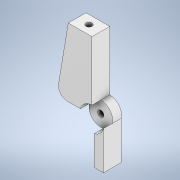
# Autodesk Inventor part: pliers
Saved by Autodesk Inventor 2020 (Build 240168000, 168)
## iProperties
Created: 2019-12-24
Part Number: pliers
Material: ABS Plastic
Document SubType Name: Modeling
Designer: metal
Density: 1.06 g/cm^3
Appearance: Smooth - White
Author: metal
Autodesk Inventor part; units mm, degrees
ref_plane "YZ Plane" through (0, 0, 0) normal (1, 0, 0) x (0, 1, 0)
ref_plane "XZ Plane" through (0, 0, 0) normal (0, 1, 0) x (-1, 0, 0)
ref_plane "XY Plane" through (0, 0, 0) normal (0, 0, 1) x (1, 0, 0)
sketch "Sketch1" plane through (0, 0, 0) normal (0, 0, 1) x (1, 0, 0)
  circle A0 centre (0, 0) radius 4
  line L0 (0, 24) -> (-8, 24)
  line L1 (0, 24) -> (0, 4)
  line L2 (-11.873, 1) -> (-3.873, 1)
  line L3 (-11.873, 1) -> (-8, 24)
  dimension "d0" = 8
  dimension "d6" = 8
  dimension "d60" = 20
  dimension "d61" = 8
  constraints: 8 end point, 2 horizontal, 2 point on circle, 1 centre point, 1 coincident, 1 vertical
  measures "d0" diameter of A0
  measures "d6" distance of L0.start L0.end
  measures "d60" distance of L0.start L1.end
  measures "d61" distance of L2.start L2.end
extrude "Extrusion1" add sketch "Sketch1" along normal mid plane 6
sketch "Sketch2" plane through (0, 0, 3) normal (0, 0, 1) x (1, 0, 0)
  circle A0 centre (0, 0) radius 4
  constraints: 1 centre point, 1 coincident
extrude "Extrusion2" cut sketch "Sketch2" against normal blind 3
sketch "Sketch4" plane through (-8, 24, 3) normal (0, 1, 0) x (1, 0, 0)
  line L0 (8, 6) -> (8, 0) projected
  line L1 (0, 0) -> (8, 6)
  line L2 (8, 0) -> (0, 0) projected
  line L3 (0, 6) -> (0, 0) projected
  line L4 (8, 0) -> (0, 6)
  line L5 (0, 6) -> (8, 6) projected
  line L6 (4, 6) -> (4, 0)
  arc A0 (3.9001, 2.005) -> (3.9001, 3.995) centre (4, 3) ccw
  arc A1 (3.9001, 3.995) -> (3.2, 3.6) centre (4, 3) ccw
  arc A2 (3.2, 2.4) -> (3.9001, 2.005) centre (4, 3) ccw
  arc A3 (3.2, 3.6) -> (3.2, 2.4) centre (4, 3) ccw
  point P0 (8, 3)
  constraints: 8 point on circle, 6 end point, 4 centre point, 3 midpoint, 2 point on line, 1 concentric
extrude "Extrusion4" cut sketch "Sketch4" against normal blind 6 contours A0 L4 L1 | L1 L6 A0 | A0 L6 L4 | L6 A0 A2 L1 | L1 A3 L4 | L4 A1 A0 L6
sketch "Sketch8" plane through (0, 0, 0) normal (0, 0, 1) x (1, 0, 0)
  arc A0 (-3.873, 1) -> (0, 4) centre (0, 0) ccw projected
  constraints: 1 coincident
hole "Hole3" at (0, 0, 0) direction (0, 0, -1) diameter 2.1 end through all
sketch "Sketch9" plane through (0, 0, 0) normal (0, 0, 1) x (1, 0, 0)
  line L0 (0, 4) -> (0, 24) construction
  line L1 (0, 24) -> (-8, 24) construction
  line L2 (-3.2679, 22.7321) -> (-9.2774, 0.3045) construction
  line L3 (-11.873, 1) -> (-3.873, 1) construction
  arc A0 (0, 4) -> (-3.873, 1) centre (0, 0) ccw construction
  arc A1 (-3.873, 1) -> (0, 4) centre (0, 0) ccw projected
  line L4 (0, 26.7661) -> (0, -20.5966) construction
  arc A2 (-3.873, 1) -> (0, 4) centre (0, 0) ccw construction
  line L5 (0.8, -3.9192) -> (0.8, -8.9192)
  line L6 (3.9, -0.8888) -> (3.9, -5.8888)
  line L7 (3.9, -5.8888) -> (3.9, -13.8305)
  line L8 (0.8, -8.9192) -> (0.8, -13.8305)
  line L9 (0.8, -13.8305) -> (3.9, -13.8305)
  point P0 (3.9, -0.8888)
  dimension "d42" = 5
  dimension "d43" = 0.8
  dimension "d49" = 5
  dimension "d56" = 3.1
  dimension "d57" = 9.9113
  constraints: 10 end point, 4 vertical, 2 point on circle, 1 perpendicular
  measures "d42" distance of L5.start L5.end
  measures "d43" distance between parallel lines of L4 L5
  measures "d49" distance of L6.start L6.end
  measures "d56" distance between parallel lines of L5 L6
  measures "d57" distance of L5.start L8.end
extrude "Extrusion5" add sketch "Sketch9" along normal mid plane 6
sketch "Sketch10" plane through (0, 0, -3) normal (0, 0, -1) x (-1, 0, 0)
  circle A0 centre (0, 0) radius 2.1
  circle A1 centre (0, 0) radius 1.05 projected
  circle A2 centre (0, 0) radius 1.05 projected
  line L0 (0, 24) -> (0, 4) projected
  arc A3 (0, 4) -> (-3.9, -0.8888) centre (0, 0) ccw projected
  line L1 (3.873, 1) -> (11.873, 1) projected
  line L2 (8, 24) -> (0, 24) projected
  line L3 (-3.9, -0.8888) -> (-3.9, -13.8305) projected
  line L4 (-0.8, -13.8305) -> (-0.8, -3.9192) projected
  arc A4 (-0.8, -3.9192) -> (3.873, 1) centre (0, 0) ccw projected
  line L5 (-3.9, -13.8305) -> (-0.8, -13.8305) projected
  line L6 (11.873, 1) -> (8, 24) projected
  dimension "d52" = 4.2
  constraints: 1 centre point, 1 coincident
  measures "d52" diameter of A0
extrude "Extrusion6" cut sketch "Sketch10" against normal blind 1 contours A0
fillet "Fillet4" radius 3 1 edges at (-11.873, 1, 0)
body "Solid1"
